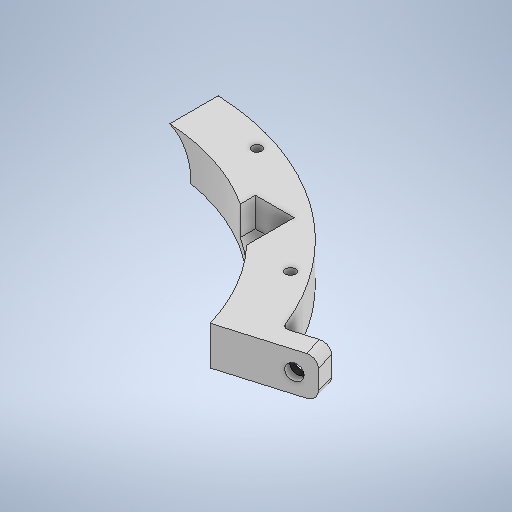
# Autodesk Inventor part: Cylinder Spacer Bottom_Q2
Saved by Autodesk Inventor 2025 (Build 290162000, 162)
## iProperties
Created: 2024-04-27
Part Number: Cylinder Spacer Bottom_Q2
Material: Generic
Document SubType Name: Modeling
Designer: Thienan Hoang
Density: 1 g/cm^3
Appearance: Default
Author: Thienan Hoang
Autodesk Inventor part; units mm, degrees
ref_plane "YZ Plane" through (0, 0, 0) normal (1, 0, 0) x (0, 1, 0)
ref_plane "XZ Plane" through (0, 0, 0) normal (0, 1, 0) x (-1, 0, 0)
ref_plane "XY Plane" through (0, 0, 0) normal (0, 0, 1) x (1, 0, 0)
sketch "Sketch1" plane through (0, 0, 0) normal (0, 1, 0) x (-1, 0, 0)
  circle A0 centre (0, 0) radius 135
  circle A1 centre (0, 0) radius 110
  dimension "d0" = 270
  dimension "d1" = 220
  constraints: 2 centre point, 2 coincident
  measures "d0" diameter of A0
  measures "d1" diameter of A1
extrude "Extrusion1" add sketch "Sketch1" along normal mid plane 47
sketch "Sketch2" plane through (0, 0, 0) normal (0, 0, 1) x (1, 0, 0)
  circle A0 centre (0, -20.5) radius 18
  line L0 (-135, -23.5) -> (135, -23.5) projected
  dimension "d4" = 36
  dimension "d38" = 3
  constraints: 1 centre point, 1 coincident
  measures "d4" diameter of A0
  measures "d38" distance from line of L0 A0.centre
extrude "Extrusion2" cut sketch "Sketch2" against normal through all
sketch "Sketch3" plane through (0, 23.5, 0) normal (0, 1, 0) x (1, 0, 0)
  circle A0 centre (0, 0) radius 127.5
  circle A1 centre (-127.5, 0) radius 2
  circle A2 centre (-103.1497, -74.9426) radius 2
  circle A3 centre (-39.3997, -121.2597) radius 2
  circle A4 centre (39.3997, -121.2597) radius 2
  circle A5 centre (103.1497, -74.9426) radius 2
  circle A6 centre (127.5, 0) radius 2
  circle A7 centre (103.1497, 74.9426) radius 2
  circle A8 centre (39.3997, 121.2597) radius 2
  circle A9 centre (-39.3997, 121.2597) radius 2
  circle A10 centre (-103.1497, 74.9426) radius 2
  dimension "d7" = 255
  dimension "d8" = 4
  dimension "d11" = 360
  constraints: 10 centre point, 1 coincident, 1 horizontal alignment, 23 other
  measures "d8" diameter of A1
hole "Hole1" at (39.3997, 23.5, 121.2597) at (-39.3997, 23.5, 121.2597) at (-103.1497, 23.5, 74.9426) at (-127.5, 23.5, 0) at (-103.1497, 23.5, -74.9426) at (-39.3997, 23.5, -121.2597) at (39.3997, 23.5, -121.2597) at (103.1497, 23.5, -74.9426) at (127.5, 23.5, 0) at (103.1497, 23.5, 74.9426) direction (0, -1, 0) diameter 5 end through all
sketch "Sketch4" plane through (0, 23.5, 0) normal (0, 1, 0) x (1, 0, 0)
  circle A0 centre (0, 0) radius 140
  constraints: 1 centre point, 1 coincident
extrude "Extrusion3" cut sketch "Sketch4" against normal blind 27
sketch "Sketch7" plane through (0, -3.5, 0) normal (0, 1, 0) x (1, 0, 0)
  line L0 (0, 0) -> (70, 0)
  line L1 (80, -100) -> (60, -100)
  line L2 (60, -100) -> (60, 100)
  line L3 (60, 100) -> (80, 100)
  line L4 (80, 100) -> (80, -100)
  line L5 (80, -100) -> (60, 100) construction
  line L6 (60, -100) -> (80, 100) construction
  dimension "d39" = 70
  dimension "d40" = 20
  dimension "d41" = 200
  constraints: 14 end point, 2 horizontal, 2 midpoint, 2 parallel, 1 perpendicular
  measures "d39" distance of L0.start L0.end
  measures "d40" distance of L2.end L3.end
  measures "d41" distance of L1.end L2.end
extrude "Extrusion7" cut sketch "Sketch7" against normal blind 15
sketch "Sketch8" plane through (0, -3.5, 0) normal (0, 1, 0) x (1, 0, 0)
  line L0 (-129.4827, -38.1999) -> (129.4827, 38.1999)
  line L1 (0, 134.8703) -> (0, -135)
  arc A0 (-5.9161, 134.8703) -> (5.9161, 134.8703) centre (0, 0) ccw projected
  constraints: 4 end point, 1 coincident, 1 midpoint
extrude "Extrusion8" cut sketch "Sketch8" against normal through all
sketch "Sketch9" plane through (0, -3.5, 0) normal (0, 1, 0) x (1, 0, 0)
  line L0 (-129.4827, -38.1999) -> (-105.5044, -31.1258) projected
  arc A0 (-5.9161, 109.8408) -> (-105.5044, -31.1258) centre (0, 0) ccw projected
  line L1 (-5.9161, 134.8703) -> (-5.9161, 109.8408) projected
  arc A1 (-5.9161, 134.8703) -> (-129.4827, -38.1999) centre (0, 0) ccw projected
  circle A2 centre (-39.3997, 121.2597) radius 2.5 projected
  circle A3 centre (-103.1497, 74.9426) radius 2.5 projected
  circle A4 centre (-127.5, 0) radius 2.5 projected
extrude "Extrusion9" cut sketch "Sketch9" against normal through all
sketch "Sketch10" plane through (129.4827, -23.5, -38.1999) normal (0.2829619, 0, 0.9591312) x (0.9591312, 0, -0.2829619)
  line L0 (0, 0) -> (-25, 0) projected
  line L1 (-2.5, 0) -> (15, 0)
  line L2 (20, 5) -> (20, 15)
  line L3 (15, 20) -> (-2.5, 20)
  line L4 (-2.5, 20) -> (-2.5, 0)
  line L5 (0, 20) -> (0, 0) projected
  arc A0 (20, 15) -> (15, 20) centre (15, 15) ccw
  arc A1 (15, 0) -> (20, 5) centre (15, 5) ccw
  point P0 (-135, 23.5)
  point P1 (20, 20)
  point P2 (20, 0)
  point P3 (0, 0)
  dimension "d48" = 22.5
  dimension "d49" = 20
  dimension "d50" = 20
  dimension "d53" = 5
  constraints: 8 end point, 5 point on line, 4 point on circle, 4 tangent, 2 centre point, 2 parallel, 1 equal radius, 1 horizontal, 1 perpendicular
  measures "d48" distance of L3.end point (20, 20)
  measures "d49" distance of point (20, 20) point (20, 0)
  measures "d50" distance between parallel lines of L5 L2
  measures "d53" radius of A0
extrude "Extrusion10" add sketch "Sketch10" against normal blind 10
fillet "Fillet1" radius 2.5 1 edges at (126.2974, -13.5, -47.6862)
sketch "Sketch11" plane through (126.6531, -23.5, -47.7912) normal (-0.2829619, 0, -0.9591312) x (-0.9591312, 0, 0.2829619)
  line L0 (-1.9306, 20) -> (-15, 20) projected
  line L1 (-20, 15) -> (-20, 5) projected
  point P0 (135, 23.5)
  point P1 (-10, 10)
  dimension "d55" = 10
  dimension "d56" = 10
  measures "d55" distance from line of L0 point (-10, 10)
  measures "d56" distance from line of L1 point (-10, 10)
hole "Hole2" at (136.2444, -13.5, -50.6208) direction (0.2829619, 0, 0.9591312) diameter 8.2 end through all counterbore diameter 13.2 counterbore depth 6
body "Solid1"
